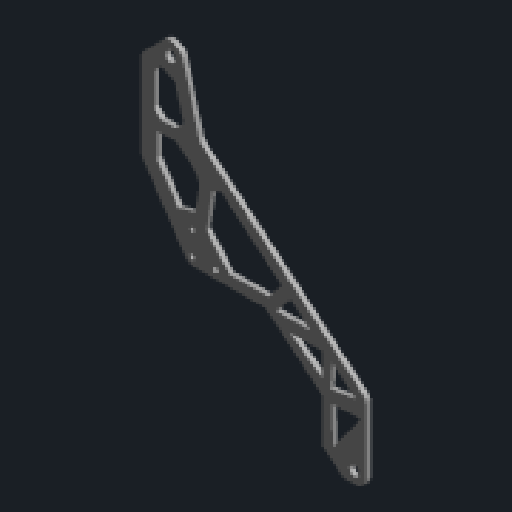
# Autodesk Inventor part: ShoulderBracketRedesign
Saved by Autodesk Inventor 2025.2 (Build 292293000, 293)
## iProperties
Created: 2025-01-19
Part Number: ShoulderBracketRedesign
Material: Generic
Document SubType Name: Sheet Metal
Designer: valer
Density: 1 g/cm^3
Sheet Metal Rule: Default
Appearance: Default
Author: valer
Autodesk Inventor part; units mm, degrees
ref_plane "YZ Plane" through (0, 0, 0) normal (1, 0, 0) x (0, 1, 0)
ref_plane "XZ Plane" through (0, 0, 0) normal (0, 1, 0) x (-1, 0, 0)
ref_plane "XY Plane" through (0, 0, 0) normal (0, 0, 1) x (1, 0, 0)
sketch "Profile" plane through (0, 0, 0) normal (0, 0, 1) x (1, 0, 0)
  circle A0 centre (-41.4125, 89.9251) radius 3.175
  circle A1 centre (-27.9037, 3.7025) radius 1.5875
  circle A2 centre (-27.8803, -10.7935) radius 1.5875
  circle A3 centre (-13.3843, -10.7935) radius 1.5875
  circle A4 centre (72.5232, -75.6183) radius 3.175
  line L0 (-43.1149, 99.546) -> (-34.6506, 95.599)
  line L1 (-34.6506, 95.599) -> (-23.2362, 53)
  line L2 (-23.2362, 53) -> (79.5232, -33.2254)
  line L3 (-43.1149, 99.546) -> (-59.4044, 83.2171)
  line L4 (-59.4044, 83.2171) -> (-59.3372, 27.6567)
  line L5 (-59.3372, 27.6567) -> (-30.5183, -15.7204)
  line L6 (-30.5183, -15.7204) -> (17.4817, -15.6624)
  line L7 (65.5232, -82.6183) -> (79.5232, -82.6183)
  line L8 (79.5232, -82.6183) -> (79.5232, -33.2254)
  line L9 (17.4817, -15.6624) -> (52.5232, -45.0657)
  line L10 (-87.1899, 0) -> (107.3087, 0) construction
  line L11 (0, -119.0512) -> (0, 135.9789) construction
  line L12 (-36.2503, -15.7274) -> (-46.8807, -15.7402) construction
  line L13 (-41.4125, 89.9251) -> (-41.2847, -15.7335) construction
  line L14 (72.5232, -75.6183) -> (72.5232, 0) construction
  line L15 (72.5232, -75.6183) -> (0, -75.6183) construction
  line L16 (-41.4125, 89.9251) -> (0, 89.9251) construction
  line L17 (-23.2362, 53) -> (-59.3372, 27.6567) construction
  line L18 (23.9517, -13.8645) -> (32.6799, -3.0672)
  line L19 (-15.6986, 30.74) -> (-10.1602, 32.89)
  line L20 (-10.1602, 32.89) -> (27.3216, 1.4391)
  line L21 (-15.6986, 30.74) -> (-19.2013, 8.0713)
  line L22 (-19.2013, 8.0713) -> (-5.274, -8.6899)
  line L23 (-5.274, -8.6899) -> (19.1575, -8.6603)
  line L24 (19.1575, -8.6603) -> (27.3216, 1.4391)
  line L25 (-25.993, 13.7438) -> (-23.435, 30.2982)
  line L26 (-23.435, 30.2982) -> (-25.4448, 35.4753)
  line L27 (-25.4448, 35.4753) -> (-37.872, 45.903)
  line L28 (-49.7674, 30.8778) -> (-36.5022, 10.9116)
  line L29 (-36.5022, 10.9116) -> (-25.993, 13.7438)
  line L30 (-49.7674, 30.8778) -> (-49.7855, 45.8886)
  line L31 (-49.7855, 45.8886) -> (-37.872, 45.903)
  line L32 (52.5232, -45.0657) -> (52.5232, -71.7101)
  line L33 (52.5232, -71.7101) -> (65.5232, -82.6183)
  line L34 (-38.6692, 52.7662) -> (-33.1987, 57.5138)
  line L35 (-33.1987, 57.5138) -> (-38.5608, 77.5256)
  line L36 (-38.5608, 77.5256) -> (-47.0549, 81.4864)
  line L37 (-47.0549, 81.4864) -> (-51.5318, 77.2647)
  line L38 (-51.5318, 77.2647) -> (-51.5078, 57.4488)
  line L39 (-51.5078, 57.4488) -> (-46.8759, 52.7563)
  line L40 (-46.8759, 52.7563) -> (-38.6692, 52.7662)
  line L41 (32.6799, -3.0672) -> (45.3602, -13.8645)
  line L42 (45.3602, -13.8645) -> (23.9517, -13.8645)
  line L43 (32.6799, -21.3341) -> (52.5232, -21.3341)
  line L44 (32.6799, -21.3341) -> (52.5232, -35.6319)
  line L45 (52.5232, -35.6319) -> (52.5232, -21.3341)
  line L46 (58.4785, -46.424) -> (59.1425, -69.4967)
  line L47 (59.1425, -69.4967) -> (76.4098, -45.908)
  line L48 (76.4098, -45.908) -> (58.4785, -46.424)
  line L49 (57.3166, -38.9544) -> (58.6445, -24.0152)
  line L50 (58.6445, -24.0152) -> (73.2517, -36.7965)
  line L51 (73.2517, -36.7965) -> (57.3166, -38.9544)
  point P0 (0, 0)
  point P1 (65.5232, -75.6183)
  point P2 (-16, 37.7902)
  point P3 (-51.3919, 28.3472)
  point P4 (-34.7148, 3.2455)
  point P5 (-52.349, 37.4497)
  point P6 (-29.1922, 43.0466)
  dimension "d0" = 7
  dimension "d1" = 7
  dimension "d3" = 8
  dimension "d4" = 8
  dimension "d5" = 8
  dimension "d6" = 65
  dimension "d7" = 15
  dimension "d8" = 45
  dimension "d12" = 145
  dimension "d17" = 18
  dimension "d37" = 35
  dimension "d56" = 53
  dimension "d63" = 7
  dimension "d65" = 120
  dimension "d66" = 7
  dimension "d68" = 20
  dimension "d69" = 48
  dimension "d70" = 4.9237
  measures "d0" distance from line of L8 L14.start
  measures "d1" distance from line of L7 L14.start
  measures "d3" distance from line of L0 L13.start
  measures "d4" distance from line of L3 L13.start
  measures "d5" distance from line of L1 L13.start
  measures "d6" angle of L11 L0
  measures "d7" angle of L11 L1
  measures "d8" angle of L13 L3
  measures "d12" angle of L1 L2
  measures "d17" distance between parallel lines of L4 L13
  measures "d37" angle of L6 L17
  measures "d56" distance from line of L10 L1.end
  measures "d63" distance between parallel lines of L18 L24
  measures "d65" angle of L19 L21
  measures "d66" distance between parallel lines of L2 L20
  measures "d68" distance between parallel lines of L14 L32
  measures "d69" distance of L5.end L6.end
  measures "d70" distance from line of L5 A2.centre
extrude "Plate1" add sketch "Profile" along normal blind 3.048
fillet "OutsideFilletsFeature" radius 6 10 edges at (65.5232, -82.6183, 1.524) (79.5232, -82.6183, 1.524) (-43.1149, 99.546, 1.524) (-34.6506, 95.599, 1.524) (-59.4044, 83.2171, 1.524) (-23.2362, 53, 1.524) (-59.3372, 27.6567, 1.524) (-30.5183, -15.7204, 1.524) (17.4817, -15.6624, 1.524) (79.5232, -33.2254, 1.524)
equation "\"d1\" = d0"
equation "\"d4\" = d3"
equation "\"d5\" = d3"
equation "\"BendRadius\" = Thickness"
equation "\"BendReliefWidth\" = Thickness"
equation "\"BendReliefDepth\" = 0.5 * Thickness"
equation "\"CornerReliefSize\" = 4 * Thickness"
equation "\"MinimumRemnant\" = 2 * Thickness"
equation "\"TransitionRadius\" = BendRadius"
equation "\"JacobiRadiusSize\" = BendRadius"
equation "\"GapSize\" = Thickness"
equation "\"Thickness\" = 3.048"
body "Solid1"
